Autodesk Inventor part; units mm, degrees
(part 2 of 2)
  spline S147 degree 2 poles (77.8545, -81.214) (77.7408, -81.3302) (77.595, -81.7281) (77.595, -81.9975) knots 0 0 0 1 2 2 2
  spline S148 degree 2 poles (77.595, -81.9975) (77.595, -82.2818) (77.7457, -82.6698) (77.8693, -82.7885) knots 0 0 0 1 2 2 2
  spline S149 degree 2 poles (77.8693, -82.7885) (77.988, -82.9046) (78.2796, -83.006) (78.4254, -83.006) knots 0 0 0 1 2 2 2
  spline S150 degree 2 poles (78.4254, -83.006) (78.5762, -83.006) (78.8506, -82.9046) (78.9445, -82.8428) knots 0 0 0 1 2 2 2
  spline S151 degree 2 poles (78.9445, -82.8428) (79.0483, -82.7811) (79.204, -82.6501) (79.2609, -82.5982) knots 0 0 0 1 2 2 2
  line L299 (79.2609, -82.5982) -> (79.3301, -82.5982)
  line L300 (79.3301, -82.5982) -> (79.3301, -83.3149)
  spline S152 degree 2 poles (79.3301, -83.3149) (79.246, -83.3545) (79.0261, -83.4533) (78.9074, -83.4879) knots 0 0 0 1 2 2 2
  spline S153 degree 2 poles (78.9074, -83.4879) (78.7641, -83.5324) (78.5144, -83.5769) (78.2969, -83.5769) knots 0 0 0 1 2 2 2
  line L301 (81.5101, -80.3317) -> (80.2965, -84.18)
  line L302 (80.2965, -84.18) -> (79.7082, -84.18)
  line L303 (79.7082, -84.18) -> (80.9193, -80.3317)
  line L304 (80.9193, -80.3317) -> (81.5101, -80.3317)
  spline S154 degree 2 poles (84.9778, -81.9926) (84.9778, -82.7341) (84.1868, -83.5819) (83.4997, -83.5819) knots 0 0 0 1 2 2 2
  spline S155 degree 2 poles (83.4997, -83.5819) (82.8101, -83.5819) (82.0242, -82.7242) (82.0242, -81.9926) knots 0 0 0 1 2 2 2
  spline S156 degree 2 poles (82.0242, -81.9926) (82.0242, -81.2585) (82.8101, -80.4033) (83.4997, -80.4033) knots 0 0 0 1 2 2 2
  spline S157 degree 2 poles (83.4997, -80.4033) (84.1868, -80.4033) (84.9778, -81.2536) (84.9778, -81.9926) knots 0 0 0 1 2 2 2
  spline S158 degree 2 poles (84.1868, -81.9926) (84.1868, -81.7182) (84.0756, -81.3351) (83.9792, -81.214) knots 0 0 0 1 2 2 2
  spline S159 degree 2 poles (83.9792, -81.214) (83.8828, -81.088) (83.6357, -80.9792) (83.5022, -80.9792) knots 0 0 0 1 2 2 2
  spline S160 degree 2 poles (83.5022, -80.9792) (83.3613, -80.9792) (83.1314, -81.0806) (83.0252, -81.2091) knots 0 0 0 1 2 2 2
  spline S161 degree 2 poles (83.0252, -81.2091) (82.9312, -81.3277) (82.8151, -81.7207) (82.8151, -81.9926) knots 0 0 0 1 2 2 2
  spline S162 degree 2 poles (82.8151, -81.9926) (82.8151, -82.2744) (82.9263, -82.6451) (83.0227, -82.7712) knots 0 0 0 1 2 2 2
  spline S163 degree 2 poles (83.0227, -82.7712) (83.1191, -82.8972) (83.3687, -83.006) (83.5022, -83.006) knots 0 0 0 1 2 2 2
  spline S164 degree 2 poles (83.5022, -83.006) (83.6381, -83.006) (83.8902, -82.8898) (83.9817, -82.7662) knots 0 0 0 1 2 2 2
  spline S165 degree 2 poles (83.9817, -82.7662) (84.0806, -82.6328) (84.1868, -82.2793) (84.1868, -81.9926) knots 0 0 0 1 2 2 2
  line L305 (63.8378, -100.2344) -> (63.0667, -103.2844)
  line L306 (63.0667, -103.2844) -> (62.2263, -103.2844)
  line L307 (62.2263, -103.2844) -> (61.737, -101.3985)
  line L308 (61.737, -101.3985) -> (61.2649, -103.2844)
  line L309 (61.2649, -103.2844) -> (60.422, -103.2844)
  line L310 (60.422, -103.2844) -> (59.6509, -100.2344)
  line L311 (59.6509, -100.2344) -> (60.4468, -100.2344)
  line L312 (60.4468, -100.2344) -> (60.8669, -102.2759)
  line L313 (60.8669, -102.2759) -> (61.3761, -100.2344)
  line L314 (61.3761, -100.2344) -> (62.1374, -100.2344)
  line L315 (62.1374, -100.2344) -> (62.6218, -102.2784)
  line L316 (62.6218, -102.2784) -> (63.0618, -100.2344)
  line L317 (63.0618, -100.2344) -> (63.8378, -100.2344)
  line L318 (63.8873, -103.2844) -> (64.918, -100.2344)
  line L319 (64.918, -100.2344) -> (65.7534, -100.2344)
  line L320 (65.7534, -100.2344) -> (66.784, -103.2844)
  line L321 (66.784, -103.2844) -> (65.9956, -103.2844)
  line L322 (65.9956, -103.2844) -> (65.8053, -102.6615)
  line L323 (65.8053, -102.6615) -> (64.8463, -102.6615)
  line L324 (64.8463, -102.6615) -> (64.6535, -103.2844)
  line L325 (64.6535, -103.2844) -> (63.8873, -103.2844)
  line L326 (65.6372, -102.1079) -> (65.3258, -101.0994)
  line L327 (65.3258, -101.0994) -> (65.0119, -102.1079)
  line L328 (65.0119, -102.1079) -> (65.6372, -102.1079)
  line L329 (69.9057, -103.2844) -> (68.9739, -103.2844)
  line L330 (68.9739, -103.2844) -> (68.1261, -102.1647)
  line L331 (68.1261, -102.1647) -> (67.8493, -102.1647)
  line L332 (67.8493, -102.1647) -> (67.8493, -103.2844)
  line L333 (67.8493, -103.2844) -> (67.0881, -103.2844)
  line L334 (67.0881, -103.2844) -> (67.0881, -100.2344)
  line L335 (67.0881, -100.2344) -> (68.314, -100.2344)
  spline S166 degree 2 poles (68.314, -100.2344) (68.5686, -100.2344) (68.9442, -100.2986) (69.1049, -100.3975) knots 0 0 0 1 2 2 2
  spline S167 degree 2 poles (69.1049, -100.3975) (69.268, -100.5013) (69.4608, -100.8251) (69.4608, -101.0723) knots 0 0 0 1 2 2 2
  spline S168 degree 2 poles (69.4608, -101.0723) (69.4608, -101.4208) (69.1445, -101.8582) (68.88, -101.9868) knots 0 0 0 1 2 2 2
  line L336 (68.88, -101.9868) -> (69.9057, -103.2844)
  spline S169 degree 2 poles (68.6748, -101.1687) (68.6748, -101.0525) (68.5859, -100.8869) (68.4845, -100.8424) knots 0 0 0 1 2 2 2
  spline S170 degree 2 poles (68.4845, -100.8424) (68.4128, -100.8127) (68.2374, -100.7954) (68.1064, -100.7954) knots 0 0 0 1 2 2 2
  line L337 (68.1064, -100.7954) -> (67.8493, -100.7954)
  line L338 (67.8493, -100.7954) -> (67.8493, -101.616)
  line L339 (67.8493, -101.616) -> (68.0693, -101.616)
  spline S171 degree 2 poles (68.0693, -101.616) (68.2275, -101.616) (68.4524, -101.5765) (68.529, -101.5147) knots 0 0 0 1 2 2 2
  spline S172 degree 2 poles (68.529, -101.5147) (68.6032, -101.4554) (68.6748, -101.2972) (68.6748, -101.1687) knots 0 0 0 1 2 2 2
  line L340 (72.7456, -103.2844) -> (72.0091, -103.2844)
  line L341 (72.0091, -103.2844) -> (70.8326, -101.1588)
  line L342 (70.8326, -101.1588) -> (70.8326, -103.2844)
  line L343 (70.8326, -103.2844) -> (70.1331, -103.2844)
  line L344 (70.1331, -103.2844) -> (70.1331, -100.2344)
  line L345 (70.1331, -100.2344) -> (71.0723, -100.2344)
  line L346 (71.0723, -100.2344) -> (72.0462, -101.9818)
  line L347 (72.0462, -101.9818) -> (72.0462, -100.2344)
  line L348 (72.0462, -100.2344) -> (72.7456, -100.2344)
  line L349 (72.7456, -100.2344) -> (72.7456, -103.2844)
  line L350 (77.4121, -103.2844) -> (76.4803, -103.2844)
  line L351 (76.4803, -103.2844) -> (75.6325, -102.1647)
  line L352 (75.6325, -102.1647) -> (75.3557, -102.1647)
  line L353 (75.3557, -102.1647) -> (75.3557, -103.2844)
  line L354 (75.3557, -103.2844) -> (74.5944, -103.2844)
  line L355 (74.5944, -103.2844) -> (74.5944, -100.2344)
  line L356 (74.5944, -100.2344) -> (75.8203, -100.2344)
  spline S173 degree 2 poles (75.8203, -100.2344) (76.0749, -100.2344) (76.4506, -100.2986) (76.6113, -100.3975) knots 0 0 0 1 2 2 2
  spline S174 degree 2 poles (76.6113, -100.3975) (76.7744, -100.5013) (76.9672, -100.8251) (76.9672, -101.0723) knots 0 0 0 1 2 2 2
  spline S175 degree 2 poles (76.9672, -101.0723) (76.9672, -101.4208) (76.6508, -101.8582) (76.3863, -101.9868) knots 0 0 0 1 2 2 2
  line L357 (76.3863, -101.9868) -> (77.4121, -103.2844)
  spline S176 degree 2 poles (76.1812, -101.1687) (76.1812, -101.0525) (76.0922, -100.8869) (75.9909, -100.8424) knots 0 0 0 1 2 2 2
  spline S177 degree 2 poles (75.9909, -100.8424) (75.9192, -100.8127) (75.7437, -100.7954) (75.6127, -100.7954) knots 0 0 0 1 2 2 2
  line L358 (75.6127, -100.7954) -> (75.3557, -100.7954)
  line L359 (75.3557, -100.7954) -> (75.3557, -101.616)
  line L360 (75.3557, -101.616) -> (75.5757, -101.616)
  spline S178 degree 2 poles (75.5757, -101.616) (75.7338, -101.616) (75.9588, -101.5765) (76.0354, -101.5147) knots 0 0 0 1 2 2 2
  spline S179 degree 2 poles (76.0354, -101.5147) (76.1095, -101.4554) (76.1812, -101.2972) (76.1812, -101.1687) knots 0 0 0 1 2 2 2
  line L361 (77.6395, -103.2844) -> (77.6395, -100.2344)
  line L362 (77.6395, -100.2344) -> (79.7008, -100.2344)
  line L363 (79.7008, -100.2344) -> (79.7008, -100.8152)
  line L364 (79.7008, -100.8152) -> (78.4007, -100.8152)
  line L365 (78.4007, -100.8152) -> (78.4007, -101.3516)
  line L366 (78.4007, -101.3516) -> (79.5995, -101.3516)
  line L367 (79.5995, -101.3516) -> (79.5995, -101.9324)
  line L368 (79.5995, -101.9324) -> (78.4007, -101.9324)
  line L369 (78.4007, -101.9324) -> (78.4007, -102.7035)
  line L370 (78.4007, -102.7035) -> (79.7008, -102.7035)
  line L371 (79.7008, -102.7035) -> (79.7008, -103.2844)
  line L372 (79.7008, -103.2844) -> (77.6395, -103.2844)
  spline S180 degree 2 poles (81.1616, -103.3388) (80.8106, -103.3388) (80.2816, -103.2028) (80.0543, -103.1039) knots 0 0 0 1 2 2 2
  line L373 (80.0543, -103.1039) -> (80.0543, -102.3773)
  line L374 (80.0543, -102.3773) -> (80.1235, -102.3773)
  spline S181 degree 2 poles (80.1235, -102.3773) (80.3533, -102.5725) (80.9045, -102.7826) (81.164, -102.7826) knots 0 0 0 1 2 2 2
  spline S182 degree 2 poles (81.164, -102.7826) (81.2308, -102.7826) (81.4458, -102.753) (81.5101, -102.7233) knots 0 0 0 1 2 2 2
  spline S183 degree 2 poles (81.5101, -102.7233) (81.5891, -102.6887) (81.7004, -102.5627) (81.7004, -102.4613) knots 0 0 0 1 2 2 2
  spline S184 degree 2 poles (81.7004, -102.4613) (81.7004, -102.3452) (81.5199, -102.2018) (81.3964, -102.1697) knots 0 0 0 1 2 2 2
  spline S185 degree 2 poles (81.3964, -102.1697) (81.2406, -102.1277) (80.8872, -102.056) (80.7315, -102.0016) knots 0 0 0 1 2 2 2
  spline S186 degree 2 poles (80.7315, -102.0016) (80.378, -101.878) (80.0716, -101.4554) (80.0716, -101.139) knots 0 0 0 1 2 2 2
  spline S187 degree 2 poles (80.0716, -101.139) (80.0716, -100.7114) (80.7957, -100.18) (81.3395, -100.18) knots 0 0 0 1 2 2 2
  spline S188 degree 2 poles (81.3395, -100.18) (81.6114, -100.18) (82.1502, -100.2912) (82.3628, -100.3851) knots 0 0 0 1 2 2 2
  line L375 (82.3628, -100.3851) -> (82.3628, -101.0821)
  line L376 (82.3628, -101.0821) -> (82.296, -101.0821)
  spline S189 degree 2 poles (82.296, -101.0821) (82.1255, -100.9363) (81.6361, -100.7361) (81.3791, -100.7361) knots 0 0 0 1 2 2 2
  spline S190 degree 2 poles (81.3791, -100.7361) (81.2777, -100.7361) (81.1195, -100.7658) (81.0306, -100.8053) knots 0 0 0 1 2 2 2
  spline S191 degree 2 poles (81.0306, -100.8053) (80.9589, -100.8375) (80.8551, -100.966) (80.8551, -101.0451) knots 0 0 0 1 2 2 2
  spline S192 degree 2 poles (80.8551, -101.0451) (80.8551, -101.1637) (81.0207, -101.2997) (81.2579, -101.354) knots 0 0 0 1 2 2 2
  spline S193 degree 2 poles (81.2579, -101.354) (81.4112, -101.3886) (81.6954, -101.4554) (81.8586, -101.5122) knots 0 0 0 1 2 2 2
  spline S194 degree 2 poles (81.8586, -101.5122) (82.1749, -101.6284) (82.4839, -102.014) (82.4839, -102.3303) knots 0 0 0 1 2 2 2
  spline S195 degree 2 poles (82.4839, -102.3303) (82.4839, -102.7851) (81.7696, -103.3388) (81.1616, -103.3388) knots 0 0 0 1 2 2 2
  line L377 (82.8769, -103.2844) -> (82.8769, -100.2344)
  line L378 (82.8769, -100.2344) -> (84.9382, -100.2344)
  line L379 (84.9382, -100.2344) -> (84.9382, -100.8152)
  line L380 (84.9382, -100.8152) -> (83.6381, -100.8152)
  line L381 (83.6381, -100.8152) -> (83.6381, -101.3516)
  line L382 (83.6381, -101.3516) -> (84.8369, -101.3516)
  line L383 (84.8369, -101.3516) -> (84.8369, -101.9324)
  line L384 (84.8369, -101.9324) -> (83.6381, -101.9324)
  line L385 (83.6381, -101.9324) -> (83.6381, -102.7035)
  line L386 (83.6381, -102.7035) -> (84.9382, -102.7035)
  line L387 (84.9382, -102.7035) -> (84.9382, -103.2844)
  line L388 (84.9382, -103.2844) -> (82.8769, -103.2844)
  line L389 (86.043, -103.2844) -> (86.043, -100.8152)
  line L390 (86.043, -100.8152) -> (85.1409, -100.8152)
  line L391 (85.1409, -100.8152) -> (85.1409, -100.2344)
  line L392 (85.1409, -100.2344) -> (87.7114, -100.2344)
  line L393 (87.7114, -100.2344) -> (87.7114, -100.8152)
  line L394 (87.7114, -100.8152) -> (86.8092, -100.8152)
  line L395 (86.8092, -100.8152) -> (86.8092, -103.2844)
  line L396 (86.8092, -103.2844) -> (86.043, -103.2844)
  line L397 (84.5791, -93.705) -> (83.8426, -93.705)
  line L398 (83.8426, -93.705) -> (82.6661, -91.5794)
  line L399 (82.6661, -91.5794) -> (82.6661, -93.705)
  line L400 (82.6661, -93.705) -> (81.9666, -93.705)
  line L401 (81.9666, -93.705) -> (81.9666, -90.655)
  line L402 (81.9666, -90.655) -> (82.9058, -90.655)
  line L403 (82.9058, -90.655) -> (83.8797, -92.4024)
  line L404 (83.8797, -92.4024) -> (83.8797, -90.655)
  line L405 (83.8797, -90.655) -> (84.5791, -90.655)
  line L406 (84.5791, -90.655) -> (84.5791, -93.705)
  spline S196 degree 2 poles (87.9752, -92.18) (87.9752, -92.9215) (87.1842, -93.7693) (86.4971, -93.7693) knots 0 0 0 1 2 2 2
  spline S197 degree 2 poles (86.4971, -93.7693) (85.8075, -93.7693) (85.0216, -92.9116) (85.0216, -92.18) knots 0 0 0 1 2 2 2
  spline S198 degree 2 poles (85.0216, -92.18) (85.0216, -91.4459) (85.8075, -90.5907) (86.4971, -90.5907) knots 0 0 0 1 2 2 2
  spline S199 degree 2 poles (86.4971, -90.5907) (87.1842, -90.5907) (87.9752, -91.441) (87.9752, -92.18) knots 0 0 0 1 2 2 2
  spline S200 degree 2 poles (87.1842, -92.18) (87.1842, -91.9056) (87.073, -91.5225) (86.9766, -91.4014) knots 0 0 0 1 2 2 2
  spline S201 degree 2 poles (86.9766, -91.4014) (86.8802, -91.2754) (86.6331, -91.1666) (86.4996, -91.1666) knots 0 0 0 1 2 2 2
  spline S202 degree 2 poles (86.4996, -91.1666) (86.3587, -91.1666) (86.1289, -91.268) (86.0226, -91.3965) knots 0 0 0 1 2 2 2
  spline S203 degree 2 poles (86.0226, -91.3965) (85.9286, -91.5151) (85.8125, -91.9081) (85.8125, -92.18) knots 0 0 0 1 2 2 2
  spline S204 degree 2 poles (85.8125, -92.18) (85.8125, -92.4618) (85.9237, -92.8325) (86.0201, -92.9586) knots 0 0 0 1 2 2 2
  spline S205 degree 2 poles (86.0201, -92.9586) (86.1165, -93.0846) (86.3661, -93.1934) (86.4996, -93.1934) knots 0 0 0 1 2 2 2
  spline S206 degree 2 poles (86.4996, -93.1934) (86.6355, -93.1934) (86.8876, -93.0772) (86.9791, -92.9536) knots 0 0 0 1 2 2 2
  spline S207 degree 2 poles (86.9791, -92.9536) (87.078, -92.8202) (87.1842, -92.4667) (87.1842, -92.18) knots 0 0 0 1 2 2 2
  line L407 (91.2476, -93.705) -> (90.3158, -93.705)
  line L408 (90.3158, -93.705) -> (89.468, -92.5853)
  line L409 (89.468, -92.5853) -> (89.1912, -92.5853)
  line L410 (89.1912, -92.5853) -> (89.1912, -93.705)
  line L411 (89.1912, -93.705) -> (88.4299, -93.705)
  line L412 (88.4299, -93.705) -> (88.4299, -90.655)
  line L413 (88.4299, -90.655) -> (89.6559, -90.655)
  spline S208 degree 2 poles (89.6559, -90.655) (89.9105, -90.655) (90.2861, -90.7193) (90.4468, -90.8181) knots 0 0 0 1 2 2 2
  spline S209 degree 2 poles (90.4468, -90.8181) (90.6099, -90.9219) (90.8027, -91.2457) (90.8027, -91.4929) knots 0 0 0 1 2 2 2
  spline S210 degree 2 poles (90.8027, -91.4929) (90.8027, -91.8414) (90.4863, -92.2789) (90.2219, -92.4074) knots 0 0 0 1 2 2 2
  line L414 (90.2219, -92.4074) -> (91.2476, -93.705)
  spline S211 degree 2 poles (90.0167, -91.5893) (90.0167, -91.4731) (89.9278, -91.3075) (89.8264, -91.263) knots 0 0 0 1 2 2 2
  spline S212 degree 2 poles (89.8264, -91.263) (89.7547, -91.2334) (89.5793, -91.2161) (89.4483, -91.2161) knots 0 0 0 1 2 2 2
  line L415 (89.4483, -91.2161) -> (89.1912, -91.2161)
  line L416 (89.1912, -91.2161) -> (89.1912, -92.0366)
  line L417 (89.1912, -92.0366) -> (89.4112, -92.0366)
  spline S213 degree 2 poles (89.4112, -92.0366) (89.5694, -92.0366) (89.7943, -91.9971) (89.8709, -91.9353) knots 0 0 0 1 2 2 2
  spline S214 degree 2 poles (89.8709, -91.9353) (89.9451, -91.876) (90.0167, -91.7178) (90.0167, -91.5893) knots 0 0 0 1 2 2 2
  line L418 (94.5893, -93.705) -> (93.828, -93.705)
  line L419 (93.828, -93.705) -> (93.828, -91.6832)
  line L420 (93.828, -91.6832) -> (93.2744, -92.9882)
  line L421 (93.2744, -92.9882) -> (92.7504, -92.9882)
  line L422 (92.7504, -92.9882) -> (92.1967, -91.6832)
  line L423 (92.1967, -91.6832) -> (92.1967, -93.705)
  line L424 (92.1967, -93.705) -> (91.475, -93.705)
  line L425 (91.475, -93.705) -> (91.475, -90.655)
  line L426 (91.475, -90.655) -> (92.3574, -90.655)
  line L427 (92.3574, -90.655) -> (93.0346, -92.1602)
  line L428 (93.0346, -92.1602) -> (93.7069, -90.655)
  line L429 (93.7069, -90.655) -> (94.5893, -90.655)
  line L430 (94.5893, -90.655) -> (94.5893, -93.705)
  line L431 (98.0129, -48.0132) -> (96.7326, -48.0132)
  line L432 (96.7326, -48.0132) -> (96.7326, -48.5891)
  line L433 (96.7326, -48.5891) -> (97.9115, -48.5891)
  line L434 (97.9115, -48.5891) -> (97.9115, -49.1699)
  line L435 (97.9115, -49.1699) -> (96.7326, -49.1699)
  line L436 (96.7326, -49.1699) -> (96.7326, -50.4824)
  line L437 (96.7326, -50.4824) -> (95.9713, -50.4824)
  line L438 (95.9713, -50.4824) -> (95.9713, -47.4324)
  line L439 (95.9713, -47.4324) -> (98.0129, -47.4324)
  line L440 (98.0129, -47.4324) -> (98.0129, -48.0132)
  line L441 (98.0055, -55.5041) -> (95.9713, -55.5041)
  line L442 (95.9713, -55.5041) -> (95.9713, -52.4541)
  line L443 (95.9713, -52.4541) -> (96.7375, -52.4541)
  line L444 (96.7375, -52.4541) -> (96.7375, -54.9233)
  line L445 (96.7375, -54.9233) -> (98.0055, -54.9233)
  line L446 (98.0055, -54.9233) -> (98.0055, -55.5041)
  line L447 (97.4889, -60.5259) -> (95.8477, -60.5259)
  line L448 (95.8477, -60.5259) -> (95.8477, -59.9945)
  line L449 (95.8477, -59.9945) -> (96.2852, -59.9945)
  line L450 (96.2852, -59.9945) -> (96.2852, -58.0073)
  line L451 (96.2852, -58.0073) -> (95.8477, -58.0073)
  line L452 (95.8477, -58.0073) -> (95.8477, -57.4759)
  line L453 (95.8477, -57.4759) -> (97.4889, -57.4759)
  line L454 (97.4889, -57.4759) -> (97.4889, -58.0073)
  line L455 (97.4889, -58.0073) -> (97.0514, -58.0073)
  line L456 (97.0514, -58.0073) -> (97.0514, -59.9945)
  line L457 (97.0514, -59.9945) -> (97.4889, -59.9945)
  line L458 (97.4889, -59.9945) -> (97.4889, -60.5259)
  line L459 (98.789, -65.5476) -> (97.8572, -65.5476)
  line L460 (97.8572, -65.5476) -> (97.0094, -64.428)
  line L461 (97.0094, -64.428) -> (96.7326, -64.428)
  line L462 (96.7326, -64.428) -> (96.7326, -65.5476)
  line L463 (96.7326, -65.5476) -> (95.9713, -65.5476)
  line L464 (95.9713, -65.5476) -> (95.9713, -62.4976)
  line L465 (95.9713, -62.4976) -> (97.1972, -62.4976)
  spline S215 degree 2 poles (97.1972, -62.4976) (97.4518, -62.4976) (97.8275, -62.5619) (97.9882, -62.6607) knots 0 0 0 1 2 2 2
  spline S216 degree 2 poles (97.9882, -62.6607) (98.1513, -62.7646) (98.3441, -63.0883) (98.3441, -63.3355) knots 0 0 0 1 2 2 2
  spline S217 degree 2 poles (98.3441, -63.3355) (98.3441, -63.684) (98.0277, -64.1215) (97.7632, -64.25) knots 0 0 0 1 2 2 2
  line L466 (97.7632, -64.25) -> (98.789, -65.5476)
  spline S218 degree 2 poles (97.5581, -63.4319) (97.5581, -63.3157) (97.4691, -63.1501) (97.3678, -63.1056) knots 0 0 0 1 2 2 2
  spline S219 degree 2 poles (97.3678, -63.1056) (97.2961, -63.076) (97.1206, -63.0587) (96.9896, -63.0587) knots 0 0 0 1 2 2 2
  line L467 (96.9896, -63.0587) -> (96.7326, -63.0587)
  line L468 (96.7326, -63.0587) -> (96.7326, -63.8793)
  line L469 (96.7326, -63.8793) -> (96.9526, -63.8793)
  spline S220 degree 2 poles (96.9526, -63.8793) (97.1107, -63.8793) (97.3357, -63.8397) (97.4123, -63.7779) knots 0 0 0 1 2 2 2
  spline S221 degree 2 poles (97.4123, -63.7779) (97.4864, -63.7186) (97.5581, -63.5604) (97.5581, -63.4319) knots 0 0 0 1 2 2 2
  spline S222 degree 2 poles (102.1245, -76.1327) (101.9243, -76.2143) (101.2841, -76.37) (100.9727, -76.37) knots 0 0 0 1 2 2 2
  spline S223 degree 2 poles (100.9727, -76.37) (100.2535, -76.37) (99.4007, -75.5395) (99.4007, -74.7783) knots 0 0 0 1 2 2 2
  spline S224 degree 2 poles (99.4007, -74.7783) (99.4007, -74.0615) (100.2535, -73.1964) (100.9949, -73.1964) knots 0 0 0 1 2 2 2
  spline S225 degree 2 poles (100.9949, -73.1964) (101.378, -73.1964) (101.8575, -73.3422) (102.1121, -73.4658) knots 0 0 0 1 2 2 2
  line L470 (102.1121, -73.4658) -> (102.1121, -74.1826)
  line L471 (102.1121, -74.1826) -> (102.0429, -74.1826)
  spline S226 degree 2 poles (102.0429, -74.1826) (101.9885, -74.1406) (101.7809, -73.9799) (101.6821, -73.9256) knots 0 0 0 1 2 2 2
  spline S227 degree 2 poles (101.6821, -73.9256) (101.5684, -73.8588) (101.2668, -73.7649) (101.0988, -73.7649) knots 0 0 0 1 2 2 2
  spline S228 degree 2 poles (101.0988, -73.7649) (100.9035, -73.7649) (100.5797, -73.8885) (100.4537, -74.0145) knots 0 0 0 1 2 2 2
  spline S229 degree 2 poles (100.4537, -74.0145) (100.3325, -74.1381) (100.1917, -74.5163) (100.1917, -74.7659) knots 0 0 0 1 2 2 2
  spline S230 degree 2 poles (100.1917, -74.7659) (100.1917, -75.2998) (100.728, -75.8089) (101.1902, -75.8089) knots 0 0 0 1 2 2 2
  spline S231 degree 2 poles (101.1902, -75.8089) (101.2322, -75.8089) (101.341, -75.804) (101.383, -75.8015) knots 0 0 0 1 2 2 2
  line L472 (101.383, -75.8015) -> (101.383, -75.2009)
  line L473 (101.383, -75.2009) -> (100.7923, -75.2009)
  line L474 (100.7923, -75.2009) -> (100.7923, -74.63)
  line L475 (100.7923, -74.63) -> (102.1245, -74.63)
  line L476 (102.1245, -74.63) -> (102.1245, -76.1327)
  line L477 (102.3741, -76.3057) -> (103.4048, -73.2557)
  line L478 (103.4048, -73.2557) -> (104.2402, -73.2557)
  line L479 (104.2402, -73.2557) -> (105.2709, -76.3057)
  line L480 (105.2709, -76.3057) -> (104.4824, -76.3057)
  line L481 (104.4824, -76.3057) -> (104.2921, -75.6829)
  line L482 (104.2921, -75.6829) -> (103.3331, -75.6829)
  line L483 (103.3331, -75.6829) -> (103.1403, -76.3057)
  line L484 (103.1403, -76.3057) -> (102.3741, -76.3057)
  line L485 (104.124, -75.1292) -> (103.8126, -74.1208)
  line L486 (103.8126, -74.1208) -> (103.4987, -75.1292)
  line L487 (103.4987, -75.1292) -> (104.124, -75.1292)
  line L488 (107.0925, -76.3057) -> (105.4513, -76.3057)
  line L489 (105.4513, -76.3057) -> (105.4513, -75.7743)
  line L490 (105.4513, -75.7743) -> (105.8888, -75.7743)
  line L491 (105.8888, -75.7743) -> (105.8888, -73.7871)
  line L492 (105.8888, -73.7871) -> (105.4513, -73.7871)
  line L493 (105.4513, -73.7871) -> (105.4513, -73.2557)
  line L494 (105.4513, -73.2557) -> (107.0925, -73.2557)
  line L495 (107.0925, -73.2557) -> (107.0925, -73.7871)
  line L496 (107.0925, -73.7871) -> (106.655, -73.7871)
  line L497 (106.655, -73.7871) -> (106.655, -75.7743)
  line L498 (106.655, -75.7743) -> (107.0925, -75.7743)
  line L499 (107.0925, -75.7743) -> (107.0925, -76.3057)
  line L500 (110.2142, -76.3057) -> (109.4776, -76.3057)
  line L501 (109.4776, -76.3057) -> (108.3011, -74.1801)
  line L502 (108.3011, -74.1801) -> (108.3011, -76.3057)
  line L503 (108.3011, -76.3057) -> (107.6016, -76.3057)
  line L504 (107.6016, -76.3057) -> (107.6016, -73.2557)
  line L505 (107.6016, -73.2557) -> (108.5409, -73.2557)
  line L506 (108.5409, -73.2557) -> (109.5147, -75.0032)
  line L507 (109.5147, -75.0032) -> (109.5147, -73.2557)
  line L508 (109.5147, -73.2557) -> (110.2142, -73.2557)
  line L509 (110.2142, -73.2557) -> (110.2142, -76.3057)
  line L510 (98.9929, -95.4843) -> (100.0236, -92.4343)
  line L511 (100.0236, -92.4343) -> (100.859, -92.4343)
  line L512 (100.859, -92.4343) -> (101.8897, -95.4843)
  line L513 (101.8897, -95.4843) -> (101.1012, -95.4843)
  line L514 (101.1012, -95.4843) -> (100.9109, -94.8614)
  line L515 (100.9109, -94.8614) -> (99.9519, -94.8614)
  line L516 (99.9519, -94.8614) -> (99.7591, -95.4843)
  line L517 (99.7591, -95.4843) -> (98.9929, -95.4843)
  line L518 (100.7428, -94.3078) -> (100.4314, -93.2993)
  line L519 (100.4314, -93.2993) -> (100.1175, -94.3078)
  line L520 (100.1175, -94.3078) -> (100.7428, -94.3078)
  spline S232 degree 2 poles (103.427, -95.5485) (102.8116, -95.5485) (102.1492, -94.9553) (102.1492, -94.3819) knots 0 0 0 1 2 2 2
  line L521 (102.1492, -94.3819) -> (102.1492, -92.4343)
  line L522 (102.1492, -92.4343) -> (102.9154, -92.4343)
  line L523 (102.9154, -92.4343) -> (102.9154, -94.3374)
  spline S233 degree 2 poles (102.9154, -94.3374) (102.9154, -94.6563) (103.1552, -94.9677) (103.427, -94.9677) knots 0 0 0 1 2 2 2
  spline S234 degree 2 poles (103.427, -94.9677) (103.6915, -94.9677) (103.9387, -94.6686) (103.9387, -94.3374) knots 0 0 0 1 2 2 2
  line L524 (103.9387, -94.3374) -> (103.9387, -92.4343)
  line L525 (103.9387, -92.4343) -> (104.7049, -92.4343)
  line L526 (104.7049, -92.4343) -> (104.7049, -94.3794)
  spline S235 degree 2 poles (104.7049, -94.3794) (104.7049, -94.943) (104.0598, -95.5485) (103.427, -95.5485) knots 0 0 0 1 2 2 2
  line L527 (105.8789, -95.4843) -> (105.8789, -93.0151)
  line L528 (105.8789, -93.0151) -> (104.9768, -93.0151)
  line L529 (104.9768, -93.0151) -> (104.9768, -92.4343)
  line L530 (104.9768, -92.4343) -> (107.5473, -92.4343)
  line L531 (107.5473, -92.4343) -> (107.5473, -93.0151)
  line L532 (107.5473, -93.0151) -> (106.6451, -93.0151)
  line L533 (106.6451, -93.0151) -> (106.6451, -95.4843)
  line L534 (106.6451, -95.4843) -> (105.8789, -95.4843)
  spline S236 degree 2 poles (110.6368, -93.9593) (110.6368, -94.7008) (109.8459, -95.5485) (109.1588, -95.5485) knots 0 0 0 1 2 2 2
  spline S237 degree 2 poles (109.1588, -95.5485) (108.4692, -95.5485) (107.6832, -94.6909) (107.6832, -93.9593) knots 0 0 0 1 2 2 2
  spline S238 degree 2 poles (107.6832, -93.9593) (107.6832, -93.2252) (108.4692, -92.37) (109.1588, -92.37) knots 0 0 0 1 2 2 2
  spline S239 degree 2 poles (109.1588, -92.37) (109.8459, -92.37) (110.6368, -93.2202) (110.6368, -93.9593) knots 0 0 0 1 2 2 2
  spline S240 degree 2 poles (109.8459, -93.9593) (109.8459, -93.6849) (109.7347, -93.3018) (109.6383, -93.1807) knots 0 0 0 1 2 2 2
  spline S241 degree 2 poles (109.6383, -93.1807) (109.5419, -93.0546) (109.2947, -92.9459) (109.1612, -92.9459) knots 0 0 0 1 2 2 2
  spline S242 degree 2 poles (109.1612, -92.9459) (109.0204, -92.9459) (108.7905, -93.0472) (108.6842, -93.1758) knots 0 0 0 1 2 2 2
  spline S243 degree 2 poles (108.6842, -93.1758) (108.5903, -93.2944) (108.4741, -93.6874) (108.4741, -93.9593) knots 0 0 0 1 2 2 2
  spline S244 degree 2 poles (108.4741, -93.9593) (108.4741, -94.241) (108.5853, -94.6118) (108.6817, -94.7378) knots 0 0 0 1 2 2 2
  spline S245 degree 2 poles (108.6817, -94.7378) (108.7781, -94.8639) (109.0278, -94.9726) (109.1612, -94.9726) knots 0 0 0 1 2 2 2
  spline S246 degree 2 poles (109.1612, -94.9726) (109.2972, -94.9726) (109.5493, -94.8565) (109.6407, -94.7329) knots 0 0 0 1 2 2 2
  spline S247 degree 2 poles (109.6407, -94.7329) (109.7396, -94.5994) (109.8459, -94.246) (109.8459, -93.9593) knots 0 0 0 1 2 2 2
  line L535 (115.2408, -85.895) -> (113.2066, -85.895)
  line L536 (113.2066, -85.895) -> (113.2066, -82.845)
  line L537 (113.2066, -82.845) -> (113.9728, -82.845)
  line L538 (113.9728, -82.845) -> (113.9728, -85.3142)
  line L539 (113.9728, -85.3142) -> (115.2408, -85.3142)
  line L540 (115.2408, -85.3142) -> (115.2408, -85.895)
  line L541 (118.1524, -82.845) -> (117.1044, -85.895)
  line L542 (117.1044, -85.895) -> (116.306, -85.895)
  line L543 (116.306, -85.895) -> (115.2581, -82.845)
  line L544 (115.2581, -82.845) -> (116.0515, -82.845)
  line L545 (116.0515, -82.845) -> (116.7163, -84.9138)
  line L546 (116.7163, -84.9138) -> (117.3787, -82.845)
  line L547 (117.3787, -82.845) -> (118.1524, -82.845)
  line L548 (120.4708, -85.895) -> (118.4366, -85.895)
  line L549 (118.4366, -85.895) -> (118.4366, -82.845)
  line L550 (118.4366, -82.845) -> (119.2028, -82.845)
  line L551 (119.2028, -82.845) -> (119.2028, -85.3142)
  line L552 (119.2028, -85.3142) -> (120.4708, -85.3142)
  line L553 (120.4708, -85.3142) -> (120.4708, -85.895)
  spline S248 degree 2 poles (117.123, -64.4708) (116.4359, -64.4708) (115.6302, -63.6403) (115.6302, -62.8889) knots 0 0 0 1 2 2 2
  spline S249 degree 2 poles (115.6302, -62.8889) (115.6302, -62.1647) (116.4384, -61.3021) (117.1255, -61.3021) knots 0 0 0 1 2 2 2
  spline S250 degree 2 poles (117.1255, -61.3021) (117.3059, -61.3021) (117.5976, -61.3441) (117.7311, -61.3788) knots 0 0 0 1 2 2 2
  spline S251 degree 2 poles (117.7311, -61.3788) (117.8349, -61.4109) (118.0796, -61.5172) (118.1562, -61.5567) knots 0 0 0 1 2 2 2
  line L554 (118.1562, -61.5567) -> (118.1562, -62.2834)
  line L555 (118.1562, -62.2834) -> (118.0796, -62.2834)
  spline S252 degree 2 poles (118.0796, -62.2834) (118.0227, -62.2339) (117.8546, -62.0955) (117.7484, -62.0313) knots 0 0 0 1 2 2 2
  spline S253 degree 2 poles (117.7484, -62.0313) (117.6421, -61.9645) (117.3875, -61.8731) (117.2466, -61.8731) knots 0 0 0 1 2 2 2
  spline S254 degree 2 poles (117.2466, -61.8731) (117.081, -61.8731) (116.8067, -61.9769) (116.6806, -62.1079) knots 0 0 0 1 2 2 2
  spline S255 degree 2 poles (116.6806, -62.1079) (116.5669, -62.2241) (116.4211, -62.622) (116.4211, -62.8914) knots 0 0 0 1 2 2 2
  spline S256 degree 2 poles (116.4211, -62.8914) (116.4211, -63.1756) (116.5719, -63.5637) (116.6954, -63.6823) knots 0 0 0 1 2 2 2
  spline S257 degree 2 poles (116.6954, -63.6823) (116.8141, -63.7985) (117.1057, -63.8998) (117.2516, -63.8998) knots 0 0 0 1 2 2 2
  spline S258 degree 2 poles (117.2516, -63.8998) (117.4023, -63.8998) (117.6767, -63.7985) (117.7706, -63.7367) knots 0 0 0 1 2 2 2
  spline S259 degree 2 poles (117.7706, -63.7367) (117.8744, -63.6749) (118.0301, -63.5439) (118.087, -63.492) knots 0 0 0 1 2 2 2
  line L556 (118.087, -63.492) -> (118.1562, -63.492)
  line L557 (118.1562, -63.492) -> (118.1562, -64.2088)
  spline S260 degree 2 poles (118.1562, -64.2088) (118.0721, -64.2483) (117.8522, -64.3472) (117.7335, -64.3818) knots 0 0 0 1 2 2 2
  spline S261 degree 2 poles (117.7335, -64.3818) (117.5902, -64.4263) (117.3405, -64.4708) (117.123, -64.4708) knots 0 0 0 1 2 2 2
  spline S262 degree 2 poles (118.5838, -67.9082) (118.5838, -68.6497) (117.7928, -69.4975) (117.1057, -69.4975) knots 0 0 0 1 2 2 2
  spline S263 degree 2 poles (117.1057, -69.4975) (116.4161, -69.4975) (115.6302, -68.6398) (115.6302, -67.9082) knots 0 0 0 1 2 2 2
  spline S264 degree 2 poles (115.6302, -67.9082) (115.6302, -67.1741) (116.4161, -66.3189) (117.1057, -66.3189) knots 0 0 0 1 2 2 2
  spline S265 degree 2 poles (117.1057, -66.3189) (117.7928, -66.3189) (118.5838, -67.1692) (118.5838, -67.9082) knots 0 0 0 1 2 2 2
  spline S266 degree 2 poles (117.7928, -67.9082) (117.7928, -67.6338) (117.6816, -67.2507) (117.5852, -67.1296) knots 0 0 0 1 2 2 2
  spline S267 degree 2 poles (117.5852, -67.1296) (117.4888, -67.0036) (117.2417, -66.8948) (117.1082, -66.8948) knots 0 0 0 1 2 2 2
  spline S268 degree 2 poles (117.1082, -66.8948) (116.9673, -66.8948) (116.7375, -66.9962) (116.6312, -67.1247) knots 0 0 0 1 2 2 2
  spline S269 degree 2 poles (116.6312, -67.1247) (116.5372, -67.2433) (116.4211, -67.6363) (116.4211, -67.9082) knots 0 0 0 1 2 2 2
  spline S270 degree 2 poles (116.4211, -67.9082) (116.4211, -68.19) (116.5323, -68.5607) (116.6287, -68.6868) knots 0 0 0 1 2 2 2
  spline S271 degree 2 poles (116.6287, -68.6868) (116.7251, -68.8128) (116.9747, -68.9216) (117.1082, -68.9216) knots 0 0 0 1 2 2 2
  spline S272 degree 2 poles (117.1082, -68.9216) (117.2441, -68.9216) (117.4962, -68.8054) (117.5877, -68.6818) knots 0 0 0 1 2 2 2
  spline S273 degree 2 poles (117.5877, -68.6818) (117.6866, -68.5484) (117.7928, -68.1949) (117.7928, -67.9082) knots 0 0 0 1 2 2 2
  line L558 (118.4206, -74.4549) -> (117.6841, -74.4549)
  line L559 (117.6841, -74.4549) -> (116.5076, -72.3293)
  line L560 (116.5076, -72.3293) -> (116.5076, -74.4549)
  line L561 (116.5076, -74.4549) -> (115.8081, -74.4549)
  line L562 (115.8081, -74.4549) -> (115.8081, -71.4049)
  line L563 (115.8081, -71.4049) -> (116.7473, -71.4049)
  line L564 (116.7473, -71.4049) -> (117.7212, -73.1524)
  line L565 (117.7212, -73.1524) -> (117.7212, -71.4049)
  line L566 (117.7212, -71.4049) -> (118.4206, -71.4049)
  line L567 (118.4206, -71.4049) -> (118.4206, -74.4549)
  line L568 (116.3939, -79.4767) -> (116.3939, -77.0075)
  line L569 (116.3939, -77.0075) -> (115.4917, -77.0075)
  line L570 (115.4917, -77.0075) -> (115.4917, -76.4267)
  line L571 (115.4917, -76.4267) -> (118.0622, -76.4267)
  line L572 (118.0622, -76.4267) -> (118.0622, -77.0075)
  line L573 (118.0622, -77.0075) -> (117.1601, -77.0075)
  line L574 (117.1601, -77.0075) -> (117.1601, -79.4767)
  line L575 (117.1601, -79.4767) -> (116.3939, -79.4767)
  spline S274 degree 2 poles (118.6776, -27.1299) (118.6776, -27.5574) (118.3044, -28.2297) (118.0202, -28.4102) knots 0 0 0 1 2 2 2
  spline S275 degree 2 poles (118.0202, -28.4102) (117.7829, -28.5634) (117.2243, -28.6524) (116.9104, -28.6524) knots 0 0 0 1 2 2 2
  line L576 (116.9104, -28.6524) -> (115.9564, -28.6524)
  line L577 (115.9564, -28.6524) -> (115.9564, -25.6024)
  line L578 (115.9564, -25.6024) -> (116.9005, -25.6024)
  spline S276 degree 2 poles (116.9005, -25.6024) (117.2218, -25.6024) (117.7829, -25.6839) (118.0301, -25.8421) knots 0 0 0 1 2 2 2
  spline S277 degree 2 poles (118.0301, -25.8421) (118.3291, -26.0349) (118.6776, -26.6874) (118.6776, -27.1299) knots 0 0 0 1 2 2 2
  spline S278 degree 2 poles (117.8917, -27.1249) (117.8917, -26.8234) (117.684, -26.3933) (117.4715, -26.2722) knots 0 0 0 1 2 2 2
  spline S279 degree 2 poles (117.4715, -26.2722) (117.3158, -26.1882) (116.9747, -26.1709) (116.7374, -26.1709) knots 0 0 0 1 2 2 2
  line L579 (116.7374, -26.1709) -> (116.7226, -26.1709)
  line L580 (116.7226, -26.1709) -> (116.7226, -28.0814)
  line L581 (116.7226, -28.0814) -> (116.7374, -28.0814)
  spline S280 degree 2 poles (116.7374, -28.0814) (116.9945, -28.0814) (117.3479, -28.0641) (117.5086, -27.9628) knots 0 0 0 1 2 2 2
  spline S281 degree 2 poles (117.5086, -27.9628) (117.6964, -27.8442) (117.8917, -27.4265) (117.8917, -27.1249) knots 0 0 0 1 2 2 2
  line L582 (115.9564, -33.6741) -> (115.9564, -30.6241)
  line L583 (115.9564, -30.6241) -> (118.0177, -30.6241)
  line L584 (118.0177, -30.6241) -> (118.0177, -31.205)
  line L585 (118.0177, -31.205) -> (116.7176, -31.205)
  line L586 (116.7176, -31.205) -> (116.7176, -31.7413)
  line L587 (116.7176, -31.7413) -> (117.9164, -31.7413)
  line L588 (117.9164, -31.7413) -> (117.9164, -32.3221)
  line L589 (117.9164, -32.3221) -> (116.7176, -32.3221)
  line L590 (116.7176, -32.3221) -> (116.7176, -33.0933)
  line L591 (116.7176, -33.0933) -> (118.0177, -33.0933)
  line L592 (118.0177, -33.0933) -> (118.0177, -33.6741)
  line L593 (118.0177, -33.6741) -> (115.9564, -33.6741)
  spline S282 degree 2 poles (118.302, -36.6073) (118.302, -36.8199) (118.166, -37.2055) (118.04, -37.334) knots 0 0 0 1 2 2 2
  spline S283 degree 2 poles (118.04, -37.334) (117.9633, -37.4156) (117.7755, -37.549) (117.6643, -37.596) knots 0 0 0 1 2 2 2
  spline S284 degree 2 poles (117.6643, -37.596) (117.5506, -37.643) (117.2861, -37.6973) (117.123, -37.6973) knots 0 0 0 1 2 2 2
  line L594 (117.123, -37.6973) -> (116.7226, -37.6973)
  line L595 (116.7226, -37.6973) -> (116.7226, -38.6959)
  line L596 (116.7226, -38.6959) -> (115.9564, -38.6959)
  line L597 (115.9564, -38.6959) -> (115.9564, -35.6459)
  line L598 (115.9564, -35.6459) -> (117.1403, -35.6459)
  spline S285 degree 2 poles (117.1403, -35.6459) (117.4023, -35.6459) (117.7854, -35.7423) (117.9411, -35.8461) knots 0 0 0 1 2 2 2
  spline S286 degree 2 poles (117.9411, -35.8461) (118.1141, -35.9622) (118.302, -36.3429) (118.302, -36.6073) knots 0 0 0 1 2 2 2
  spline S287 degree 2 poles (117.516, -36.6271) (117.516, -36.4961) (117.3924, -36.3107) (117.3084, -36.2761) knots 0 0 0 1 2 2 2
  spline S288 degree 2 poles (117.3084, -36.2761) (117.1996, -36.2292) (117.0019, -36.2143) (116.8313, -36.2143) knots 0 0 0 1 2 2 2
  line L599 (116.8313, -36.2143) -> (116.7226, -36.2143)
  line L600 (116.7226, -36.2143) -> (116.7226, -37.1289)
  line L601 (116.7226, -37.1289) -> (116.777, -37.1289)
  spline S289 degree 2 poles (116.777, -37.1289) (116.8832, -37.1289) (117.076, -37.1239) (117.1477, -37.1116) knots 0 0 0 1 2 2 2
  spline S290 degree 2 poles (117.1477, -37.1116) (117.2095, -37.1017) (117.3454, -37.0423) (117.3825, -37.0053) knots 0 0 0 1 2 2 2
  spline S291 degree 2 poles (117.3825, -37.0053) (117.4616, -36.9311) (117.516, -36.7655) (117.516, -36.6271) knots 0 0 0 1 2 2 2
  line L602 (118.774, -43.7176) -> (117.8422, -43.7176)
  line L603 (117.8422, -43.7176) -> (116.9945, -42.598)
  line L604 (116.9945, -42.598) -> (116.7176, -42.598)
  line L605 (116.7176, -42.598) -> (116.7176, -43.7176)
  line L606 (116.7176, -43.7176) -> (115.9564, -43.7176)
  line L607 (115.9564, -43.7176) -> (115.9564, -40.6676)
  line L608 (115.9564, -40.6676) -> (117.1823, -40.6676)
  spline S292 degree 2 poles (117.1823, -40.6676) (117.4369, -40.6676) (117.8126, -40.7319) (117.9732, -40.8307) knots 0 0 0 1 2 2 2
  spline S293 degree 2 poles (117.9732, -40.8307) (118.1364, -40.9346) (118.3291, -41.2583) (118.3291, -41.5055) knots 0 0 0 1 2 2 2
  spline S294 degree 2 poles (118.3291, -41.5055) (118.3291, -41.854) (118.0128, -42.2915) (117.7483, -42.42) knots 0 0 0 1 2 2 2
  line L609 (117.7483, -42.42) -> (118.774, -43.7176)
  spline S295 degree 2 poles (117.5432, -41.6019) (117.5432, -41.4857) (117.4542, -41.3201) (117.3528, -41.2756) knots 0 0 0 1 2 2 2
  spline S296 degree 2 poles (117.3528, -41.2756) (117.2812, -41.246) (117.1057, -41.2287) (116.9747, -41.2287) knots 0 0 0 1 2 2 2
  line L610 (116.9747, -41.2287) -> (116.7176, -41.2287)
  line L611 (116.7176, -41.2287) -> (116.7176, -42.0493)
  line L612 (116.7176, -42.0493) -> (116.9376, -42.0493)
  spline S297 degree 2 poles (116.9376, -42.0493) (117.0958, -42.0493) (117.3207, -42.0097) (117.3973, -41.9479) knots 0 0 0 1 2 2 2
  spline S298 degree 2 poles (117.3973, -41.9479) (117.4715, -41.8886) (117.5432, -41.7304) (117.5432, -41.6019) knots 0 0 0 1 2 2 2
  line L613 (114.774, -31.1633) -> (113.8422, -31.1633)
  line L614 (113.8422, -31.1633) -> (112.9945, -30.0436)
  line L615 (112.9945, -30.0436) -> (112.7176, -30.0436)
  line L616 (112.7176, -30.0436) -> (112.7176, -31.1633)
  line L617 (112.7176, -31.1633) -> (111.9564, -31.1633)
  line L618 (111.9564, -31.1633) -> (111.9564, -28.1133)
  line L619 (111.9564, -28.1133) -> (113.1823, -28.1133)
  spline S299 degree 2 poles (113.1823, -28.1133) (113.4369, -28.1133) (113.8126, -28.1775) (113.9732, -28.2764) knots 0 0 0 1 2 2 2
  spline S300 degree 2 poles (113.9732, -28.2764) (114.1364, -28.3802) (114.3291, -28.704) (114.3291, -28.9511) knots 0 0 0 1 2 2 2
  spline S301 degree 2 poles (114.3291, -28.9511) (114.3291, -29.2996) (114.0128, -29.7371) (113.7483, -29.8656) knots 0 0 0 1 2 2 2
  line L620 (113.7483, -29.8656) -> (114.774, -31.1633)
  spline S302 degree 2 poles (113.5432, -29.0475) (113.5432, -28.9314) (113.4542, -28.7658) (113.3528, -28.7213) knots 0 0 0 1 2 2 2
  spline S303 degree 2 poles (113.3528, -28.7213) (113.2812, -28.6916) (113.1057, -28.6743) (112.9747, -28.6743) knots 0 0 0 1 2 2 2
  line L621 (112.9747, -28.6743) -> (112.7176, -28.6743)
  line L622 (112.7176, -28.6743) -> (112.7176, -29.4949)
  line L623 (112.7176, -29.4949) -> (112.9376, -29.4949)
  spline S304 degree 2 poles (112.9376, -29.4949) (113.0958, -29.4949) (113.3207, -29.4554) (113.3973, -29.3936) knots 0 0 0 1 2 2 2
  spline S305 degree 2 poles (113.3973, -29.3936) (113.4715, -29.3342) (113.5432, -29.1761) (113.5432, -29.0475) knots 0 0 0 1 2 2 2
  line L624 (111.9564, -36.185) -> (111.9564, -33.135)
  line L625 (111.9564, -33.135) -> (114.0177, -33.135)
  line L626 (114.0177, -33.135) -> (114.0177, -33.7158)
  line L627 (114.0177, -33.7158) -> (112.7176, -33.7158)
  line L628 (112.7176, -33.7158) -> (112.7176, -34.2522)
  line L629 (112.7176, -34.2522) -> (113.9164, -34.2522)
  line L630 (113.9164, -34.2522) -> (113.9164, -34.833)
  line L631 (113.9164, -34.833) -> (112.7176, -34.833)
  line L632 (112.7176, -34.833) -> (112.7176, -35.6042)
  line L633 (112.7176, -35.6042) -> (114.0177, -35.6042)
  line L634 (114.0177, -35.6042) -> (114.0177, -36.185)
  line L635 (114.0177, -36.185) -> (111.9564, -36.185)
  line L636 (112.5421, -41.2067) -> (112.5421, -38.7376)
  line L637 (112.5421, -38.7376) -> (111.64, -38.7376)
  line L638 (111.64, -38.7376) -> (111.64, -38.1567)
  line L639 (111.64, -38.1567) -> (114.2105, -38.1567)
  line L640 (114.2105, -38.1567) -> (114.2105, -38.7376)
  line L641 (114.2105, -38.7376) -> (113.3084, -38.7376)
  line L642 (113.3084, -38.7376) -> (113.3084, -41.2067)
  line L643 (113.3084, -41.2067) -> (112.5421, -41.2067)
  point P0 (0, 0)
  point P1 (5, -30.45)
  point P2 (5, -30.45)
  point P3 (5, -49.47)
  point P4 (5, -68.49)
  point P5 (5, -49.47)
  point P6 (5, -68.49)
  point P7 (-4.5, -53)
  point P8 (-4.5, -59.5)
  point P9 (-9, -53)
  point P10 (-4.5, -53)
  point P11 (4.9824, -85.6324)
  point P12 (73.6502, -100.18)
  point P13 (73.6502, -84.18)
  point P14 (98.7, -56.49)
  point P15 (111.64, -34.66)
  point P16 (115.64, -34.66)
  dimension "d78" = 8
  dimension "d79" = 8
  dimension "d80" = 8
  dimension "d81" = 8
  dimension "d82" = 8
  dimension "d83" = 8
  dimension "d84" = 8
  dimension "d85" = 8
  constraints: 18 end point, 13 midpoint, 4 horizontal, 3 vertical, 2 point on line, 1 perpendicular, 34 other
  measures "d78" distance of L75.start L75.end
  measures "d79" distance of L75.start L76.end
  measures "d80" distance of L77.start L77.end
  measures "d81" distance of L77.start L78.end
  measures "d82" distance of L77.start L79.end
  measures "d83" distance of L80.start L80.end
  measures "d84" distance of L80.start L81.end
  measures "d85" distance of L80.start L82.end
extrude "Extrusion5" add sketch "Sketch3" along normal blind 0.9
sketch "Sketch4" plane through (0, 0, 3.5) normal (0, 0, 1) x (1, 0, 0)
  line L0 (23.08, -25.88) -> (23.08, -35.02) projected
  arc A0 (23.08, -25.88) -> (21.08, -23.88) centre (21.08, -25.88) ccw projected
  line L1 (12, -23.88) -> (21.08, -23.88) projected
  arc A1 (12, -23.88) -> (10, -25.88) centre (12, -25.88) ccw projected
  line L2 (10, -35.02) -> (10, -25.88) projected
  arc A2 (10, -35.02) -> (12, -37.02) centre (12, -35.02) ccw projected
  line L3 (21.08, -37.02) -> (12, -37.02) projected
  arc A3 (21.08, -37.02) -> (23.08, -35.02) centre (21.08, -35.02) ccw projected
  point P0 (0, 0)
  dimension "d91" = 13.08
  measures "d91" distance between parallel lines of L0 L2
sketch "Sketch5" plane through (0, 0, 3.5) normal (0, 0, 1) x (1, 0, 0)
  line L0 (0, -59.5) -> (0, -97) projected
  line L1 (-9, -59.5) -> (0, -59.5) projected
  line L2 (-9, -46.5) -> (-9, -59.5) projected
  line L3 (0, -46.5) -> (-9, -46.5) projected
  line L4 (0, -18) -> (0, -46.5) projected
  line L5 (0, -9) -> (0, -18) projected
  line L6 (0, -9) -> (-9, -9) projected
  line L7 (-9, -9) -> (-9, 0) projected
  line L8 (-9, 0) -> (3.5, 0) projected
  line L9 (117.3502, 0) -> (3.5, 0) projected
  line L10 (117.3502, 0) -> (129.8502, 0) projected
  line L11 (129.8502, 0) -> (129.8502, -9) projected
  line L12 (129.8502, -9) -> (120.8502, -9) projected
  line L13 (120.8502, -18) -> (120.8502, -9) projected
  line L14 (120.8502, -46.5) -> (120.8502, -18) projected
  line L15 (129.8502, -46.5) -> (120.8502, -46.5) projected
  line L16 (129.8502, -59.5) -> (129.8502, -46.5) projected
  line L17 (120.8502, -59.5) -> (129.8502, -59.5) projected
  line L18 (120.8502, -97) -> (120.8502, -59.5) projected
  line L19 (120.8502, -97) -> (129.8502, -97) projected
  line L20 (129.8502, -97) -> (129.8502, -106) projected
  line L21 (129.8502, -106) -> (117.3502, -106) projected
  line L22 (3.5, -106) -> (117.3502, -106) projected
  line L23 (3.5, -106) -> (-9, -106) projected
  line L24 (-9, -106) -> (-9, -97) projected
  line L25 (-9, -97) -> (0, -97) projected
  circle A0 centre (-4.5, -101.5) radius 1.65 projected
  circle A1 centre (125.3502, -101.5) radius 1.65 projected
  circle A2 centre (125.3502, -4.5) radius 1.65 projected
  circle A3 centre (-4.5, -4.5) radius 1.65 projected
  point P0 (0, 0)
body "Solid1"
